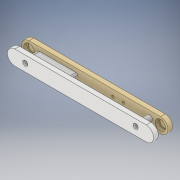
# Autodesk Inventor part: Thigh
Saved by Autodesk Inventor 2019.1 (Build 231200000, 200)
## iProperties
Created: 2018-10-31
Part Number: Thigh
Material: Generisch
Document SubType Name: Modeling
Designer: JochenAlt
Density: 1 g/cm^3
Appearance: Vorgabe
Author: JochenAlt
Autodesk Inventor part; units mm, degrees
ref_plane "YZ Plane" through (0, 0, 0) normal (1, 0, 0) x (0, 1, 0)
ref_plane "XZ Plane" through (0, 0, 0) normal (0, 1, 0) x (-1, 0, 0)
ref_plane "XY Plane" through (0, 0, 0) normal (0, 0, 1) x (1, 0, 0)
sketch "Skizze1" plane through (0, 0, 0) normal (0, 0, 1) x (1, 0, 0)
  circle A0 centre (0, 0) radius 5
  circle A1 centre (124.473, 0) radius 5
  line L0 (0, 7) -> (124.473, 7)
  line L1 (0, -7) -> (124.473, -7)
  line L2 (0, 9.8) -> (0, -9.8) construction
  line L3 (-34.6946, 0) -> (159.1676, 0) construction
  circle A2 centre (0, 0) radius 7
  circle A3 centre (124.473, 0) radius 7
  circle A4 centre (0, 0) radius 4
  circle A5 centre (124.473, 0) radius 4
  arc A6 (9.9923, 3.25) -> (10.2168, -2.4545) centre (9.9923, 0.3933) ccw
  circle A7 centre (9.9923, 0.3933) radius 1.2
  circle A8 centre (114.473, 0.8929) radius 1.2
  circle A9 centre (9.9923, 0.3933) radius 2.4
  circle A10 centre (114.473, 0.8929) radius 2.4
  line L4 (10.2168, -2.4545) -> (44.5759, 0.2546)
  line L5 (44.458, 3.25) -> (9.9923, 3.25)
  circle A11 centre (89.473, 1) radius 1.2
  circle A12 centre (89.473, 1) radius 1 construction
  circle A13 centre (124.473, 0) radius 4.25 construction
  circle A14 centre (0, 0) radius 4.25 construction
  line L6 (89.6511, 1.984) -> (123.716, -4.182) construction
  line L7 (124.473, 4.25) -> (0, 4.25) construction
  line L8 (89.473, 3.125) -> (124.473, 0) construction
  line L9 (89.473, 3.125) -> (89.473, 4.25) construction
  line L10 (89.473, 3.125) -> (89.473, 2) construction
  arc A15 (44.5759, 0.2546) -> (44.458, 3.25) centre (44.458, 1.75) ccw
  circle A16 centre (114.473, 0.8929) radius 2.3571
  line L11 (114.473, 3.25) -> (114.473, 4.25) construction
  circle A17 centre (79.473, 1) radius 1 construction
  circle A18 centre (79.473, 1) radius 1.2
  line L12 (89.473, 1) -> (79.473, 1) construction
  line L13 (0.3341, -4.2369) -> (79.3944, 1.9969) construction
  line L14 (79.473, 2) -> (89.473, 2) construction
  line L15 (9.9923, 0.3933) -> (44.458, 1.75) construction
  circle A19 centre (84.473, -4) radius 1.2
  line L16 (84.5613, -5.1967) -> (84.5613, -7) construction
  line L17 (80.3215, 0.1515) -> (83.6245, -3.1515) construction
  line L18 (85.3215, -3.1515) -> (88.6245, 0.1515) construction
  dimension "d27" = 2.4
  dimension "d0" = 10
  dimension "d2" = 124.473
  dimension "d3" = 2
  dimension "d6" = 1
  dimension "d17" = 10
  dimension "d18" = 2.4
  dimension "d20" = 4.8
  dimension "d29" = 35
  dimension "d32" = 8
  dimension "d33" = 2
  dimension "d34" = 8.5
  dimension "d38" = 1
  dimension "d39" = 10
  dimension "d40" = 1
  dimension "d41" = 10
  dimension "d42" = 1.5
  constraints: 34 end point, 19 point on circle, 17 centre point, 14 tangent, 12 coincident, 7 equal radius, 7 point on line, 3 perpendicular, 2 equal length, 2 horizontal, 2 line through centre, 2 parallel, 2 vertical, 1 collinear, 1 vertical alignment, 12 other
  measures "d0" diameter of A0
  measures "d2" distance of A1.centre point (0, 0)
  measures "d3" radial gap between concentric circles of A2 A0
  measures "d6" radial gap between concentric circles of A0 A4
  measures "d17" distance of A6.centre point (0, 0)
  measures "d18" diameter of A7
  measures "d20" diameter of A9
  measures "d29" horizontal distance of point (89.473, 1) A1.centre
  measures "d32" distance from line of L1 point (89.473, 1)
  measures "d33" diameter of A12
  measures "d34" diameter of A14
  measures "d38" distance of L11.start L11.end
  measures "d39" distance of L12.start L12.end
  measures "d40" distance between parallel lines of L7 L5
  measures "d41" horizontal distance of A1.centre A8.centre
  measures "d42" radius of A15
extrude "Extrusion1" add sketch "Skizze1" along normal blind 7.5 contours L0 A3 L1 A2 | A2 | A3 | L5 A15 L4 A6 | A9 | A10 | A16
extrude "Extrusion2" add sketch "Skizze1" along normal blind 0.5 from surface at 7.5 contours A0 | A1 | L0 A3 L1 A2 | A2 | A3 | L5 A15 L4 A6 | A7 | A8 | A9 | A10 | A16 | A19
extrude "Extrusion3" cut sketch "Skizze1" along normal blind 4.5 contours L0 A3 L1 A2 | A2 | A3 | L5 A15 L4 A6 | A7 | A8 | A9 | A10 | A11 | A16 | A18 | A19
extrude "Extrusion4" add sketch "Skizze1" along normal blind 1 from surface at 8 contours A0 | A1 | L0 A3 L1 A2 | A2 | A3 | A4 | A5 | L5 A15 L4 A6 | A9 | A10 | A11 | A16 | A18 | A19
extrude "Extrusion5" cut sketch "Skizze1" against normal blind 1.8 from surface at 9 contours A7 | A8 | A9 | A10 | A16
mirror "Spiegeln1" about plane through (0, 0, 0) normal (0, 0, 1) bodies 1 separate body
extrude "Extrusion6" add sketch "Skizze1" against normal up to surface (9 mm away) from surface at 4.5 contours L5 A15 L4 A6 | A9 | A10 | A16 bodies 1
